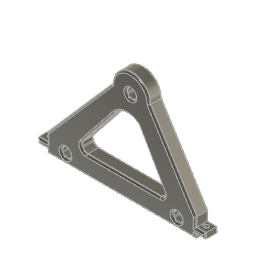
_Tape Side Walls.54dce662-5c7d-447c-ae04-a9adc093dbb2 (Autodesk Fusion 360 design; units mm, degrees)
Autodesk Fusion 360 part; units mm, degrees
sketch "Sketch1" plane through (0, 0, 0) normal (0, 0, 1) x (1, 0, 0)
  line L0 (0, 0) -> (-101.6, 0)
  line L1 (-101.6, 0) -> (-101.6, 31.75)
  line L2 (-101.6, 31.75) -> (0, 31.75)
  line L3 (0, 31.75) -> (0, 0)
  line L4 (-101.6, 0) -> (-88.9, 0)
  line L5 (-88.9, 0) -> (-88.9, -25.4)
  line L6 (-88.9, -25.4) -> (-101.6, -25.4)
  line L7 (-101.6, -25.4) -> (-101.6, 0)
  line L8 (0, 0) -> (-12.7, 0)
  line L9 (-12.7, 0) -> (-12.7, -25.4)
  line L10 (-12.7, -25.4) -> (0, -25.4)
  line L11 (0, -25.4) -> (0, 0)
  circle A0 centre (-95.25, -19.05) radius 6.35
  circle A1 centre (-6.35, -19.05) radius 6.35
  circle A2 centre (-95.25, -19.05) radius 1.5875
  circle A3 centre (-6.35, -19.05) radius 1.5875
  dimension "d1" = 101.6
  dimension "d2" = 31.75
  dimension "d3" = 12.7
  dimension "d4" = 25.4
  dimension "d5" = 12.7
  dimension "d6" = 25.4
  dimension "d7" = 3.175
  dimension "d8" = 3.175
  constraint horizontal L0
  constraint vertical L1
  constraint horizontal L2
  constraint vertical L3
  constraint coincident L0.start L3.end
  constraint horizontal L4
  constraint vertical L5
  constraint horizontal L6
  constraint vertical L7
  constraint horizontal L8
  constraint vertical L9
  constraint horizontal L10
  constraint vertical L11
  constraint tangent L7 A0
  constraint tangent L6 A0
  constraint tangent L5 A0
  constraint tangent L9 A1
  constraint tangent L10 A1
  constraint tangent L11 A1
  constraint concentric A0 A2
  constraint concentric A1 A3
  measures "d1" distance of L0.start L0.end
  measures "d2" distance of L0.start L2.end
  measures "d3" distance of L0.end L4.end
  measures "d4" distance of L0.end L6.end
  measures "d5" distance of L0.start L8.end
  measures "d6" distance of L0.start L10.end
  measures "d7" diameter of A2
  measures "d8" diameter of A3
sketch "Sketch2" plane through (0, 0, 0) normal (0, -1, 0) x (1, 0, 0)
sketch "Sketch3" plane through (0, 0, 0) normal (0, 1, 0) x (1, 0, 0)
  line L0 (0, 0) -> (-101.6, 0)
  line L1 (-101.6, 0) -> (-101.6, -63.5)
  line L2 (-101.6, -63.5) -> (0, -63.5)
  line L3 (0, -63.5) -> (0, 0)
  line L4 (0, -63.5) -> (-44.45, -63.5)
  circle A0 centre (-44.45, -63.5) radius 12.7
  circle A1 centre (-44.45, -63.5) radius 3.175
  line L5 (-101.6, 0) -> (0, 0)
  line L6 (0, 0) -> (0, -12.7)
  line L7 (0, -12.7) -> (-101.6, -12.7)
  line L8 (-101.6, -12.7) -> (-101.6, 0)
  line L9 (-101.6, -12.7) -> (-57.15, -63.5)
  line L10 (-31.75, -63.5) -> (0, -12.7)
  line L11 (-101.6, -12.7) -> (-82.55, -12.7)
  line L12 (0, -12.7) -> (-19.05, -12.7)
  line L13 (-82.55, -12.7) -> (-50.8, -52.5015)
  line L14 (-19.05, -12.7) -> (-41.0315, -51.2687)
  arc A2 (-54.6861, -47.6299) -> (-39.2079, -48.069) centre (-46.712, -39.5655) ccw
  arc A3 (-74.5793, -12.7) -> (-77.8677, -18.5696) centre (-74.5793, -16.556) ccw
  arc A4 (-21.2476, -16.556) -> (-23.9349, -12.7) centre (-23.9349, -15.5644) ccw
  line L15 (-101.6, 0) -> (-88.9, 0)
  line L16 (-88.9, 0) -> (-88.9, -6.35)
  line L17 (0, 0) -> (-12.7, 0)
  line L18 (-12.7, 0) -> (-12.7, -6.35)
  circle A5 centre (-88.9, -6.35) radius 3.175
  circle A6 centre (-12.7, -6.35) radius 3.175
  dimension "d12" = 101.6
  dimension "d13" = 63.5
  dimension "d14" = 44.45
  dimension "d15" = 25.4
  dimension "d16" = 6.35
  dimension "d17" = 12.7
  dimension "d18" = 19.05
  dimension "d19" = 19.05
  dimension "d20" = 12.7
  dimension "d21" = 6.35
  dimension "d22" = 12.7
  dimension "d23" = 6.35
  dimension "d24" = 6.35
  dimension "d25" = 6.35
  constraint horizontal L0
  constraint vertical L1
  constraint horizontal L2
  constraint vertical L3
  constraint coincident L0.start L3.end
  constraint coincident L2 L4.end
  constraint coincident L4.end A0.centre
  constraint concentric A0 A1
  constraint horizontal L5
  constraint vertical L6
  constraint horizontal L7
  constraint vertical L8
  constraint coincident A0 L9.end
  constraint coincident L2 L9.end
  constraint coincident A0 L10.start
  constraint coincident L2 L10.start
  constraint perpendicular L8 L11
  constraint perpendicular L3 L12
  constraint coincident A0 L13.end
  constraint coincident A0 L14.end
  constraint tangent A0 A2
  constraint coincident L14 A2.end
  constraint coincident L13 A2.start
  constraint tangent L7 A3
  constraint coincident L7 A3.start
  constraint coincident L13 A3.end
  constraint tangent L7 A4
  constraint coincident L7 A4.end
  constraint coincident L14 A4.start
  constraint perpendicular L8 L15
  constraint perpendicular L15 L16
  constraint perpendicular L3 L17
  constraint perpendicular L0 L18
  constraint coincident L16.end A5.centre
  constraint coincident L18.end A6.centre
  measures "d12" distance of L0.start L0.end
  measures "d13" distance of L0.start L2.end
  measures "d14" distance of L2.end L4.end
  measures "d15" diameter of A0
  measures "d16" diameter of A1
  measures "d17" distance of L0.end L7.end
  measures "d18" distance of L7.end L11.end
  measures "d19" distance of L6.end L12.end
  measures "d20" distance of L0.end L15.end
  measures "d21" distance of L15.end L16.end
  measures "d22" distance of L0.start L17.end
  measures "d23" distance of L17.end L18.end
  measures "d24" diameter of A5
  measures "d25" diameter of A6
extrude "Extrude2" add sketch "Sketch3" along normal blind 9.525 contours L0 L1 L3 L5 L6 L7 L8 L11 L12 L15 L17 | A0 L7 L10 L12 L14 | L7 L14 A4 | L2 L4 A0 A1 | L2 L4 A0 A1 | A0 L14 A2 | A0 L7 L9 L11 L13 | L7 L13 A3 | A0 L13 A2
sketch "Sketch4" plane through (0, 0, 0) normal (0, 0, 1) x (1, 0, 0)
  line L0 (0, 9.525) -> (6.35, 9.525)
  line L1 (6.35, 9.525) -> (6.35, 0)
  line L2 (6.35, 0) -> (0, 0)
  line L3 (0, 0) -> (0, 9.525)
  line L4 (-101.6, 0) -> (-101.6, 0)
  line L5 (-101.6, 0) -> (-101.6, 9.525)
  line L6 (-101.6, 9.525) -> (-101.6, 9.525)
  line L7 (-101.6, 9.525) -> (-101.6, 0)
  line L8 (-101.6, 0) -> (-107.95, 0)
  line L9 (-107.95, 0) -> (-107.95, 9.525)
  line L10 (-107.95, 9.525) -> (-101.6, 9.525)
  line L11 (-101.6, 9.525) -> (-101.6, 0)
  dimension "d28" = 6.35
  dimension "d29" = 6.35
  dimension "d30" = 9.525
  constraint horizontal L0
  constraint vertical L1
  constraint horizontal L2
  constraint vertical L3
  constraint vertical L5
  constraint vertical L7
  constraint horizontal L8
  constraint vertical L9
  constraint horizontal L10
  constraint vertical L11
  measures "d28" distance of L0.start L0.end
  measures "d29" distance of L4.start L8.end
  measures "d30" distance of L4.start L5.end
extrude "Extrude3" add sketch "Sketch4" along normal blind 6.35 and the other way blind -2.54
sketch "Sketch5" plane through (0, 0, 6.35) normal (0, 0, 1) x (-1, 0, 0)
  line L0 (101.6, -9.525) -> (107.95, -9.525)
  line L1 (107.95, -9.525) -> (107.95, 0)
  line L2 (107.95, 0) -> (101.6, 0)
  line L3 (101.6, 0) -> (101.6, -9.525)
  circle A0 centre (104.14, -5.08) radius 1.5875
  circle A1 centre (-2.54, -5.08) radius 1.5875
  dimension "d35" = 3.175
  dimension "d36" = 3.175
  measures "d35" diameter of A0
  measures "d36" diameter of A1
extrude "Extrude4" cut sketch "Sketch5" against normal blind 6.35 contours A0 | A1
fillet "Fillet1" radius 1.27 4 faces at (-17.6659, 0, 30.9187) (-17.6659, 9.525, 30.9187) (2.1167, 9.525, 3.81) (-105.8333, 9.525, 3.81)
